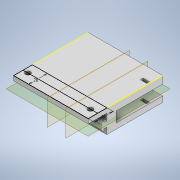
# Autodesk Inventor part: 포토게이트 설치 부분
Saved by Autodesk Inventor 2022 (Build 260153000, 153)
## iProperties
Created: 2024-01-09
Part Number: 포토게이트 설치 부분
Material: 일반
Document SubType Name: Modeling
Designer: slskz
Density: 1 g/cm^3
Appearance: 기본값
Author: slskz
Autodesk Inventor part; units mm, degrees
ref_plane "YZ Plane" through (0, 0, 0) normal (1, 0, 0) x (0, 1, 0)
ref_plane "XZ Plane" through (0, 0, 0) normal (0, 1, 0) x (-1, 0, 0)
ref_plane "XY Plane" through (0, 0, 0) normal (0, 0, 1) x (1, 0, 0)
sketch "스케치1" plane through (0, 0, 0) normal (0, 1, 0) x (-1, 0, 0)
  point P0 (0, 0)
sketch "스케치2" plane through (0, 0, 0) normal (0, 1, 0) x (-1, 0, 0)
  line L0 (-40, 40) -> (40, 40)
  line L1 (40, 40) -> (40, -40)
  line L2 (40, -40) -> (-40, -40)
  line L3 (-40, -40) -> (-40, 40)
  line L4 (-40, 40) -> (40, -40) construction
  line L5 (40, 40) -> (-40, -40) construction
  point P0 (0, 0)
  dimension "d0" = 80
  dimension "d1" = 80
  constraints: 12 end point, 2 midpoint, 2 parallel, 1 horizontal, 1 perpendicular
  measures "d0" distance of L1.end L2.end
  measures "d1" distance of L0.end L1.end
extrude "돌출1" add sketch "스케치2" along normal blind 25
sketch "스케치3" plane through (0, 0, 0) normal (0, -1, 0) x (1, 0, 0)
  point P0 (0, 0)
ref_plane "작업 평면1" through (0, 12.5, 0) normal (0, -1, 0) x (1, 0, 0)
sketch "스케치4" plane through (0, 12.5, 0) normal (0, -1, 0) x (1, 0, 0)
  point P0 (0, 0)
sketch "스케치5" plane through (0, 25, 0) normal (0, 1, 0) x (1, 0, 0)
  line L0 (-40, 40) -> (-40, -40) projected
  line L1 (-40, -20) -> (40, -20)
  line L2 (40, -40) -> (40, 40) projected
  point P0 (0, 0)
  dimension "d4" = 20
  constraints: 2 end point, 2 point on line, 1 horizontal
  measures "d4" distance of L0.end L1.start
sketch "스케치6" plane through (0, 25, 0) normal (0, 1, 0) x (1, 0, 0)
  line L0 (-40, 40) -> (-40, -40) projected
  line L1 (40, -40) -> (40, 40) projected
  line L2 (-40, -40) -> (40, -40)
  line L3 (40, -40) -> (40, -20)
  line L4 (40, -20) -> (-40, -20)
  line L5 (-40, -20) -> (-40, -40)
  line L6 (40, -30) -> (-40, -30)
  point P0 (0, 0)
  dimension "d5" = 20
  constraints: 10 end point, 2 midpoint, 2 parallel, 1 horizontal, 1 perpendicular, 1 point on line
  measures "d5" distance of L3.end L2.end
sketch "스케치7" plane through (40, 0, 40) normal (1, 0, 0) x (0, 0, -1)
  line L0 (0, 0) -> (20, 0)
  line L1 (20, 0) -> (20, 20)
  line L2 (20, 20) -> (0, 20)
  line L3 (0, 20) -> (0, 0)
  line L4 (0, 25) -> (80, 25) projected
  line L5 (20, 13) -> (17, 13)
  line L6 (20, 7) -> (17, 7)
  line L7 (17, 13) -> (17, 15)
  line L8 (17, 7) -> (17, 5)
  line L9 (17, 5) -> (16, 5)
  line L10 (17, 15) -> (16, 15)
  line L11 (14, 12.5341) -> (14, 7.5341)
  line L12 (14, 12.5341) -> (16, 15)
  line L13 (14, 7.5341) -> (16, 5)
  line L14 (0, 0) -> (0, 25) projected
  point P0 (40, 0)
  dimension "d24" = 3
  dimension "d25" = 7
  dimension "d26" = 3
  dimension "d27" = 7
  dimension "d28" = 2
  dimension "d29" = 2
  dimension "d30" = 1
  dimension "d31" = 1
  dimension "d32" = 5
  dimension "d33" = 2
  constraints: 26 end point, 4 horizontal, 3 vertical, 2 parallel, 2 perpendicular, 2 point on line
  measures "d24" distance of L5.start L5.end
  measures "d25" distance between parallel lines of L5 L2
  measures "d26" distance of L6.start L6.end
  measures "d27" distance between parallel lines of L0 L6
  measures "d28" distance of L5.end L7.end
  measures "d29" distance of L6.end L8.end
  measures "d30" distance of L8.end L9.end
  measures "d31" distance of L7.end L10.end
  measures "d32" distance of L11.start L11.end
  measures "d33" distance from line of L11 L9.end
sketch "스케치8" plane through (40, 0, 40) normal (1, 0, 0) x (0, 0, -1)
  point P0 (40, 0)
ref_plane "작업 평면2" through (0, 0, 40) normal (1, 0, 0) x (0, 0, -1)
extrude "돌출2" cut sketch "스케치7" against normal through all contours L3 L2 L1 L5 L7 L10 L12 L11 L13 L9 L8 L6 L0
ref_plane "작업 평면3" through (20, 0, -40) normal (1, 0, 0) x (0, 0, -1)
sketch "스케치10" plane through (40, 0, -40) normal (1, 0, 0) x (0, 0, -1)
  point P0 (-40, 0)
sketch "스케치11" plane through (20, 0, -40) normal (1, 0, 0) x (0, 0, -1)
  line L0 (-40, 24.3345) -> (-37.4364, 0)
  point P0 (-40, 0)
  constraints: 2 end point
sketch "스케치12" plane through (40, 0, -40) normal (1, 0, 0) x (0, 0, -1)
  line L0 (-50, 17) -> (0, 17)
  line L1 (0, 17) -> (0, 6)
  line L2 (0, 6) -> (-50, 6)
  line L3 (-50, 6) -> (-50, 17)
  line L4 (0, 0) -> (0, 25) projected
  line L5 (-80, 25) -> (0, 25) projected
  point P0 (-40, 0)
  dimension "d37" = 50
  dimension "d38" = 11
  dimension "d39" = 0
  dimension "d40" = 8
  constraints: 8 end point, 2 parallel, 1 horizontal, 1 perpendicular
  measures "d37" distance of L1.end L2.end
  measures "d38" distance of L0.end L1.end
  measures "d39" distance between parallel lines of L4 L1
  measures "d40" distance between parallel lines of L0 L5
extrude "돌출3" cut sketch "스케치12" against normal blind 16
sketch "스케치14" plane through (20, 0, -40) normal (1, 0, 0) x (0, 0, -1)
  point P0 (-40, 0)
sketch "스케치15" plane through (0, 25, 0) normal (0, 1, 0) x (1, 0, 0)
  point P0 (0, 0)
sketch "스케치16" plane through (0, 25, 0) normal (0, 1, 0) x (1, 0, 0)
  point P0 (0, 0)
  point P1 (32.6349, -30.1509)
  point P2 (-34.5495, -30.0157)
hole "구멍2" at (-34.5495, 25, 30.0157) at (32.6349, 25, 30.1509) direction (0, -1, 0) diameter 5.5 end through all clearance for "Hex Head Cap Screw" size "M5" standard "Ansi Metric M Profile"
sketch "스케치17" plane through (0, 25, 0) normal (0, 1, 0) x (1, 0, 0)
  point P0 (0, 0)
sketch "스케치19" plane through (0, 25, 0) normal (0, 1, 0) x (1, 0, 0)
  point P0 (0, 0)
sketch "스케치20" plane through (0, 25, 0) normal (0, 1, 0) x (1, 0, 0)
  line L0 (24, 40) -> (40, 40) projected
  line L1 (40, 40) -> (32, 40)
  line L2 (32, 40) -> (32, 24)
  line L3 (32, 24) -> (40, 24)
  line L4 (40, 24) -> (40, 40)
  line L5 (40, 27) -> (32, 27)
  line L6 (38.742, 24) -> (38.742, 27)
  point P0 (0, 0)
  dimension "d62" = 16
  dimension "d63" = 8
  dimension "d64" = 3
  dimension "d65" = 1.258
  constraints: 12 end point, 4 point on line, 3 perpendicular, 2 parallel, 1 horizontal
  measures "d62" distance of L2.end L1.end
  measures "d63" distance of L2.end L3.end
  measures "d64" distance of L5.end L2.end
  measures "d65" distance between parallel lines of L6 L4
extrude "돌출5" cut sketch "스케치20" against normal through all contours L5 L6 L3 L2
